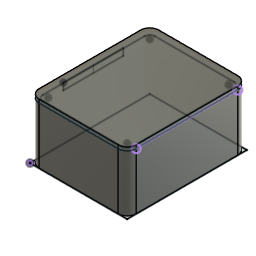
Fusion360 Norm Box Template (Autodesk Fusion 360 design; units mm, degrees)
Autodesk Fusion 360 part; units mm, degrees
sketch "Base" plane through (0, 0, 0) normal (0, 1, 0) x (1, 0, 0) in component "Case"
  line L0 (0, 0) -> (43, 0)
  line L1 (43, 0) -> (43, 53)
  line L2 (43, 53) -> (0, 53)
  line L3 (0, 53) -> (0, 0)
  dimension "d6" = 43
  dimension "d7" = 53
  constraint horizontal L0
  constraint vertical L1
  constraint horizontal L2
  constraint vertical L3
  constraint coincident L0.start L3.end
  measures "d6" distance of L0.start L0.end
  measures "d7" distance of L0.start L2.end
extrude "Extrude1" add sketch "Base" along normal blind 25 makes body 1 in component "Case"
fillet "Fillet1" radius 4 4 edges at (43, 12.5, 0) (0, 12.5, 0) (43, 12.5, -53) (0, 12.5, -53) on bodies 1 in component "Case"
shell "Shell1" thickness 1.5 removed faces 1 at (14.3333, 25, -34) on bodies 1 in component "Case"
sketch "Knob" plane through (1.5, 0, 0) normal (1, 0, 0) x (0, 0, -1) in component "Case"
  line L0 (49, 1.5) -> (49, 25)
  line L1 (49, 25) -> (4, 25)
  line L2 (4, 25) -> (4, 1.5)
  line L3 (4, 1.5) -> (49, 1.5)
  line L4 (13.25, 25) -> (39.75, 25)
  line L5 (39.75, 25) -> (39.75, 22)
  line L6 (39.75, 22) -> (13.25, 22)
  line L7 (13.25, 22) -> (13.25, 25)
  line L8 (26.5, 25) -> (26.5, 22) construction
  dimension "d12" = 26.5
  dimension "d13" = 3
  constraint horizontal L4
  constraint vertical L5
  constraint horizontal L6
  constraint vertical L7
  constraint coincident L1 L4.start
  constraint midpoint L1 L8.start
  constraint midpoint L6 L8.end
  constraint vertical L8
  measures "d12" distance of L5.end L6.end
  measures "d13" distance of L4.end L5.end
extrude "Extrude2" add sketch "Knob" along normal blind 6 draft -45 contours L1 L4 L5 L6 L7 bodies 1 in component "Case"
ref_plane "WorkPlane2" through (21.5, 12.5, -26.5) normal (-1, 0, 0) x (0, 0, 1) in component "Case"
mirror "Mirror1" about plane through (21.5, 12.5, -26.5) normal (-1, 0, 0) of "Extrude2" in component "Case"
sketch "Top" plane through (0, 25, 0) normal (0, 1, 0) x (-1, 0, 0) in component "Top Cover"
  line L0 (-43, -4) -> (-43, -49)
  arc A0 (-43, -49) -> (-39, -53) centre (-39, -49) ccw
  line L1 (-39, -53) -> (-4, -53)
  arc A1 (-4, -53) -> (0, -49) centre (-4, -49) ccw
  line L2 (0, -49) -> (0, -4)
  arc A2 (0, -4) -> (-4, 0) centre (-4, -4) ccw
  line L3 (-4, 0) -> (-39, 0)
  arc A3 (-39, 0) -> (-43, -4) centre (-39, -4) ccw
  line L4 (-41.5, -13.25) -> (-41.5, -4)
  arc A4 (-39, -1.5) -> (-41.5, -4) centre (-39, -4) ccw
  line L5 (-39, -1.5) -> (-4, -1.5)
  arc A5 (-1.5, -4) -> (-4, -1.5) centre (-4, -4) ccw
  line L6 (-1.5, -4) -> (-1.5, -13.25)
  line L7 (-1.5, -13.25) -> (-1.5, -39.75)
  line L8 (-1.5, -39.75) -> (-1.5, -49)
  arc A6 (-4, -51.5) -> (-1.5, -49) centre (-4, -49) ccw
  line L9 (-4, -51.5) -> (-39, -51.5)
  arc A7 (-41.5, -49) -> (-39, -51.5) centre (-39, -49) ccw
  line L10 (-41.5, -49) -> (-41.5, -39.75)
  line L11 (-41.5, -39.75) -> (-41.5, -13.25)
extrude "Extrude1'" add sketch "Top" along normal blind 1.5 separate body contours L0 A0 L1 A1 L2 A2 L3 A3 | L4 A4 L5 A5 L6 L7 L8 A6 L9 A7 L10 L11 makes body 2 in component "Top Cover"
sketch "Lip" plane through (0, 25, 0) normal (0, -1, 0) x (1, 0, 0) in component "Top Cover"
  arc A0 (43, -4) -> (39, 0) centre (39, -4) ccw
  line L0 (39, 0) -> (4, 0)
  arc A1 (4, 0) -> (0, -4) centre (4, -4) ccw
  line L1 (0, -4) -> (0, -49)
  arc A2 (0, -49) -> (4, -53) centre (4, -49) ccw
  line L2 (4, -53) -> (39, -53)
  arc A3 (39, -53) -> (43, -49) centre (39, -49) ccw
  line L3 (43, -49) -> (43, -4)
  line L4 (41.3, -49) -> (41.3, -4)
  arc A4 (41.3, -4) -> (39, -1.7) centre (39, -4) ccw
  line L5 (39, -1.7) -> (4, -1.7)
  arc A5 (4, -1.7) -> (1.7, -4) centre (4, -4) ccw
  line L6 (1.7, -4) -> (1.7, -49)
  arc A6 (1.7, -49) -> (4, -51.3) centre (4, -49) ccw
  line L7 (4, -51.3) -> (39, -51.3)
  arc A7 (39, -51.3) -> (41.3, -49) centre (39, -49) ccw
  line L8 (43, -4) -> (43, -49)
  dimension "d19" = 1.7
  dimension "d31" = 1.7
  measures "d31" distance of L4 L8
extrude "Extrude2'" add sketch "Lip" along normal blind 3 contours L4 A4 L5 A5 L6 A6 L7 A7 bodies 2 in component "Top Cover"
extrude "Extrude3" cut sketch "Knob" along normal blind 3 draft -45 from surface at 0.2 contours L1 L4 L5 L6 L7 bodies 2 in component "Top Cover"
ref_plane "WorkPlane2" through (21.5, 0, 0) normal (1, 0, 0) x (0, 1, 0) in component "Top Cover"
mirror "Mirror1'" about plane through (21.5, 0, 0) normal (1, 0, 0) of "Extrude3" in component "Top Cover"
shell "Shell1'" thickness 1.5 removed faces 1 at (28.1, 22, -30.9167) on bodies 2 in component "Top Cover"
chamfer "Chamfer1" distance 0.6 angle 45 2 edges at (1.7, 22, -26.5) (41.3, 22, -26.5) on bodies 2 in component "Top Cover"
component "Enclosure" placed x (1, 0, 0) y (0, 1, 0) z (0, 0, 1) at (0, 0, 0)
component "Case" placed x (1, 0, 0) y (0, 1, 0) z (0, 0, 1) at (0, 0, 0) in component "Enclosure"
component "Top Cover" placed x (1, 0, 0) y (0, 1, 0) z (0, 0, 1) at (0, 0, 0) in component "Enclosure"
equation "Width = Width_internal + ( 2 * shell )"
equation "length = Length_internal + ( 2 * shell )"
equation "heigth = 25 mm"
equation "shell = 1.5 mm"
equation "gap = 0.2 mm"
equation "d6 = length"
equation "d7 = Width"
equation "d8 = heigth"
equation "d11 = shell"
equation "d12 = Width / 2"
equation "d13 = shell * 2"
equation "d17 = shell"
equation "d19 = shell + gap"
equation "d20 = shell * 2"
equation "d23 = shell * 2"
equation "d26 = shell"
equation "d33 = length / 2"
equation "Width_internal = 50 mm"
equation "Length_internal = 40 mm"
